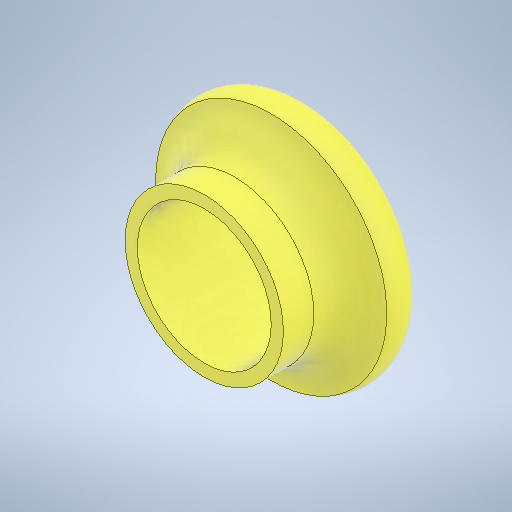
# Autodesk Inventor part: 132 part 2
Saved by Autodesk Inventor 2025.1 (Build 291241000, 241)
## iProperties
Created: 2024-08-01
Part Number: 132 part 2
Material: Steel, Alloy
Document SubType Name: Modeling
Designer: ffogue
Density: 7.73 g/cm^3
Appearance: Smooth - Yellow
Author: ffogue
Autodesk Inventor part; units mm, degrees
ref_plane "YZ Plane" through (0, 0, 0) normal (1, 0, 0) x (0, 1, 0)
ref_plane "XZ Plane" through (0, 0, 0) normal (0, 1, 0) x (-1, 0, 0)
ref_plane "XY Plane" through (0, 0, 0) normal (0, 0, 1) x (1, 0, 0)
sketch "Sketch1" plane through (0, 0, 0) normal (0, 0, 1) x (1, 0, 0)
  line L0 (0, 0) -> (-13, 0)
  line L1 (-13, 0) -> (-13, 5)
  arc A0 (-13, 5) -> (-19, 11) centre (-19, 5) ccw
  arc A1 (-15.5359, 17) -> (-19, 11) centre (-15.5359, 13) ccw
  line L2 (-15.5359, 17) -> (0, 17)
  line L3 (0, 17) -> (0, 0)
  point P0 (-19, 15)
  dimension "d0" = 4
  dimension "d1" = 6
  dimension "d2" = 38
  dimension "d3" = 11
  dimension "d4" = 26
  dimension "d13" = 6
  constraints: 8 end point, 5 point on circle, 2 centre point, 2 horizontal, 2 perpendicular, 2 tangent, 1 vertical alignment
  measures "d0" radius of A1
  measures "d1" radius of A0
  measures "d2" diameter of point (-19, 15) L3
  measures "d3" vertical distance of L0.end A0.end
  measures "d4" diameter of L0.end L3
  measures "d13" distance from line of A0.end L2
revolve "Revolution1" add sketch "Sketch1" angle 360 about axis through (0, 17, 0) along (0, -1, 0)
sketch "Sketch2" plane through (0, 0, 0) normal (0, -1, 0) x (1, 0, 0)
  circle A0 centre (0, 0) radius 13 projected
  point P0 (0, 0)
  constraints: 1 coincident
hole "Hole1" at (0, 0, 0) direction (0, 1, 0) diameter 22 depth 17
body "Solid1"
